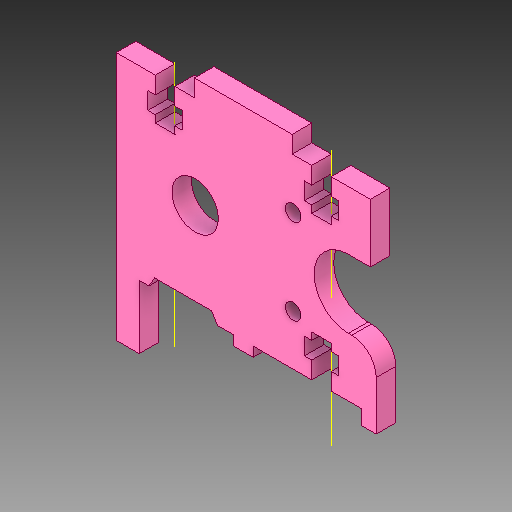
# Autodesk Inventor part: Motorhalter_rechts
Saved by Autodesk Inventor 2019 (Build 230136000, 136)
## iProperties
Created: 2022-10-31
Part Number: Motorhalter_rechts
Material: Generisch
Document SubType Name: Modeling
Designer: RP
Density: 1 g/cm^3
Appearance: Pink
Author: RP
Autodesk Inventor part; units mm, degrees
ref_plane "YZ Plane" through (0, 0, 0) normal (1, 0, 0) x (0, 1, 0)
ref_plane "XZ Plane" through (0, 0, 0) normal (0, 1, 0) x (-1, 0, 0)
ref_plane "XY Plane" through (0, 0, 0) normal (0, 0, 1) x (1, 0, 0)
sketch "Skizze1" plane through (0, 0, 0) normal (0, 0, 1) x (1, 0, 0)
  circle A0 centre (-60.768, 178.1277) radius 4.75
  circle A1 centre (-40.718, 169.3777) radius 1.6
  circle A2 centre (-40.718, 186.8777) radius 1.6
  line L0 (-23.718, 156.1277) -> (-23.718, 166.1277)
  arc A3 (-23.718, 166.1277) -> (-28.718, 171.1277) centre (-28.718, 166.1277) ccw
  line L1 (-28.718, 171.1277) -> (-29.418, 171.1277)
  arc A4 (-29.418, 185.1277) -> (-29.418, 171.1277) centre (-29.418, 178.1277) ccw
  line L2 (-40.918, 197.1277) -> (-40.918, 200.6277)
  line L3 (-40.918, 200.6277) -> (-60.918, 200.6277)
  line L4 (-68.918, 197.1277) -> (-76.918, 197.1277)
  line L5 (-76.918, 197.1277) -> (-76.918, 146.1277)
  line L6 (-76.918, 146.1277) -> (-72.218, 146.1277)
  line L7 (-72.218, 146.1277) -> (-72.218, 159.1277)
  line L8 (-72.218, 159.1277) -> (-70.218, 159.1277)
  line L9 (-70.218, 159.1277) -> (-69.0633, 161.1277)
  line L10 (-69.0633, 161.1277) -> (-57.3727, 161.1277)
  line L11 (-57.3727, 161.1277) -> (-56.218, 159.1277)
  line L12 (-56.218, 159.1277) -> (-36.918, 159.1277)
  line L13 (-32.918, 159.1277) -> (-26.718, 159.1277)
  line L14 (-26.718, 159.1277) -> (-26.718, 156.1277)
  line L15 (-26.718, 156.1277) -> (-23.718, 156.1277)
  line L16 (-36.5327, 178.1277) -> (-65.518, 178.1277) construction
  line L17 (-40.718, 169.3777) -> (-40.718, 186.8777) construction
  line L18 (-32.918, 159.1277) -> (-32.918, 162.6277)
  line L19 (-32.918, 162.6277) -> (-31.418, 162.6277)
  line L20 (-31.418, 162.6277) -> (-31.418, 166.1277)
  line L21 (-31.418, 166.1277) -> (-32.918, 166.1277)
  line L22 (-32.918, 166.1277) -> (-32.918, 167.6277)
  line L23 (-32.918, 167.6277) -> (-36.918, 167.6277)
  line L24 (-36.918, 167.6277) -> (-36.918, 166.1277)
  line L25 (-36.918, 166.1277) -> (-38.418, 166.1277)
  line L26 (-38.418, 166.1277) -> (-38.418, 162.6277)
  line L27 (-38.418, 162.6277) -> (-36.918, 162.6277)
  line L28 (-36.918, 159.1277) -> (-36.918, 162.6277)
  line L29 (-34.918, 158.3124) -> (-34.918, 166.072) construction
  line L30 (-32.918, 197.1277) -> (-32.918, 193.6277)
  line L31 (-32.918, 193.6277) -> (-31.418, 193.6277)
  line L32 (-31.418, 193.6277) -> (-31.418, 190.1277)
  line L33 (-31.418, 190.1277) -> (-32.918, 190.1277)
  line L34 (-32.918, 190.1277) -> (-32.918, 188.6277)
  line L35 (-32.918, 188.6277) -> (-36.918, 188.6277)
  line L36 (-36.918, 188.6277) -> (-36.918, 190.1277)
  line L37 (-36.918, 190.1277) -> (-38.418, 190.1277)
  line L38 (-38.418, 190.1277) -> (-38.418, 193.6277)
  line L39 (-38.418, 193.6277) -> (-36.918, 193.6277)
  line L40 (-36.918, 197.1277) -> (-36.918, 193.6277)
  line L41 (-34.918, 197.9429) -> (-34.918, 190.1833) construction
  line L42 (-32.918, 197.1277) -> (-24.918, 197.1277)
  line L43 (-50.918, 190.3199) -> (-50.918, 199.5586) construction
  line L44 (-68.918, 190.1277) -> (-68.918, 188.6277)
  line L45 (-66.918, 197.9429) -> (-66.918, 190.1833) construction
  line L46 (-64.918, 197.1277) -> (-64.918, 193.6277)
  line L47 (-68.918, 188.6277) -> (-64.918, 188.6277)
  line L48 (-63.418, 193.6277) -> (-64.918, 193.6277)
  line L49 (-63.418, 190.1277) -> (-63.418, 193.6277)
  line L50 (-64.918, 188.6277) -> (-64.918, 190.1277)
  line L51 (-64.918, 190.1277) -> (-63.418, 190.1277)
  line L52 (-70.418, 190.1277) -> (-68.918, 190.1277)
  line L53 (-68.918, 193.6277) -> (-70.418, 193.6277)
  line L54 (-70.418, 193.6277) -> (-70.418, 190.1277)
  line L55 (-68.918, 197.1277) -> (-68.918, 193.6277)
  line L56 (-29.418, 185.1277) -> (-24.918, 185.1277)
  line L57 (-24.918, 185.1277) -> (-24.918, 197.1277)
  line L58 (-60.918, 200.6277) -> (-60.918, 197.1277)
  line L59 (-36.918, 197.1277) -> (-40.918, 197.1277)
  line L60 (-60.918, 197.1277) -> (-64.918, 197.1277)
  point P0 (0, 0)
  point P1 (-40.718, 178.1277)
  point P2 (-23.718, 190.1277)
  point P3 (-28.718, 190.1277)
  point P4 (-73.118, 190.1277)
  dimension "d1" = 19
  dimension "d2" = 2
  dimension "d4" = 14
  dimension "d5" = 3
  dimension "d6" = 3
  dimension "d7" = 5
  dimension "d8" = 7
  dimension "d9" = 4.3
  dimension "d14" = 5.8
  dimension "d15" = 4
  dimension "d16" = 7
  dimension "d17" = 3.5
  dimension "d18" = 3.5
  dimension "d19" = 1.5
  dimension "d22" = 2
  dimension "d23" = 31.5
  dimension "d24" = 14
  dimension "d25" = 60
  dimension "d27" = 32
  dimension "d28" = 10
  dimension "d30" = 13
  dimension "d31" = 10
  dimension "d33" = 20
  dimension "d34" = 3.5
  constraints: 122 end point, 31 symmetric about line, 26 point on line, 15 perpendicular, 7 vertical, 5 point on circle, 4 centre point, 4 tangent, 3 horizontal, 2 collinear, 2 parallel, 1 equal length, 1 horizontal alignment, 1 midpoint, 12 other
  measures "d1" distance between parallel lines of L13 L16
  measures "d2" distance between parallel lines of L12 L10
  measures "d4" distance between parallel lines of L14 L17
  measures "d5" distance of L14.end L0.start
  measures "d6" distance between parallel lines of L13 L15
  measures "d7" radius of A3
  measures "d8" distance between parallel lines of L1 L16
  measures "d9" distance edge to line of A4 L17
  measures "d14" distance between parallel lines of L17 L29
  measures "d15" distance between parallel lines of L28 L18
  measures "d16" distance between parallel lines of L20 L26
  measures "d17" distance of L13.start L18.end
  measures "d18" distance of L19.end L20.end
  measures "d19" distance of L21.end L22.end
  measures "d22" distance of L7.end L8.end
  measures "d23" distance between parallel lines of L17 L7
  measures "d24" distance of L11.end L8.end
  measures "d25" angle of L11 L12
  measures "d27" distance between parallel lines of L45 L41
  measures "d28" distance between parallel lines of L57 L41
  measures "d30" distance between parallel lines of L8 L6
  measures "d31" distance between parallel lines of L45 L5
  measures "d33" distance of L2.end L3.end
  measures "d34" distance of L3.end L58.end
extrude "Extrusion1" add sketch "Skizze1" along normal mid plane 4
sketch "Skizze2" plane through (-56.218, 159.1277, 2) normal (0, -1, 0) x (1, 0, 0)
  line L0 (-4.7, -4) -> (15.3, -4) projected
  line L1 (15.3, 0) -> (-4.7, 0) projected
  line L2 (3.3, -4) -> (7.3, -4)
  line L3 (7.3, -4) -> (7.3, 0)
  line L4 (7.3, 0) -> (3.3, 0)
  line L5 (3.3, 0) -> (3.3, -4)
  line L6 (32.5, 0) -> (32.5, -4) projected
  point P0 (56.218, -2)
  dimension "d37" = 25.2
  dimension "d38" = 4
  constraints: 8 end point, 2 parallel, 2 point on line, 1 horizontal, 1 perpendicular
  measures "d37" distance between parallel lines of L6 L3
  measures "d38" distance between parallel lines of L3 L5
extrude "Extrusion2" add sketch "Skizze2" along normal blind 2
